Autodesk Fusion 360 part; units mm, degrees
(part 7 of 13)
  line L5346 (136.758, -112.613) -> (136.728, -112.622)
  line L5347 (137.072, -110.779) -> (137.074, -110.771)
  line L5348 (135.676, -113.181) -> (135.176, -113.181)
  line L5349 (137.072, -111.929) -> (137.072, -110.779)
  line L5350 (135.676, -111.686) -> (135.75, -111.686)
  line L5351 (137.084, -110.76) -> (137.092, -110.759)
  line L5352 (138.11, -110.76) -> (138.116, -110.765)
  line L5353 (135.176, -111.681) -> (135.676, -111.681)
  line L5354 (135.676, -111.681) -> (135.676, -111.686)
  line L5355 (138.02, -113.004) -> (137.897, -113.024)
  line L5356 (137.078, -110.765) -> (137.084, -110.76)
  line L5357 (138.12, -110.771) -> (138.122, -110.779)
  line L5358 (137.46, -110.76) -> (137.466, -110.765)
  line L5359 (137.393, -111.982) -> (137.392, -111.988)
  line L5360 (137.36, -112.041) -> (136.817, -112.585)
  line L5361 (137.392, -111.988) -> (137.375, -112.014)
  line L5362 (135.738, -113.177) -> (135.676, -113.176)
  line L5363 (136.156, -112.041) -> (136.176, -112.181)
  line L5364 (137.099, -111.949) -> (137.092, -111.949)
  line L5365 (135.996, -113.066) -> (135.875, -113.14)
  line L5366 (137.092, -110.759) -> (137.452, -110.759)
  line L5367 (135.886, -111.727) -> (136.005, -111.804)
  line L5368 (135.176, -113.181) -> (135.176, -111.681)
  line L5369 (137.472, -110.779) -> (137.472, -111.929)
  line L5370 (136.176, -112.693) -> (136.153, -112.833)
  line L5371 (136.091, -112.961) -> (135.996, -113.066)
  line L5372 (137.452, -110.759) -> (137.46, -110.76)
  line L5373 (138.116, -110.765) -> (138.12, -110.771)
  line L5374 (136.793, -112.603) -> (136.788, -112.606)
  line L5375 (135.875, -113.14) -> (135.738, -113.177)
  line L5376 (136.005, -111.804) -> (136.098, -111.912)
  line L5377 (137.074, -111.936) -> (137.072, -111.929)
  line L5378 (137.092, -111.949) -> (137.084, -111.947)
  line L5379 (137.078, -111.943) -> (137.074, -111.936)
  line L5380 (136.153, -112.833) -> (136.091, -112.961)
  line L5381 (136.176, -112.181) -> (136.176, -112.372)
  line L5382 (136.176, -112.372) -> (136.676, -112.372)
  line L5383 (141.061, -112.902) -> (140.561, -112.902)
  line L5384 (138.116, -111.943) -> (138.11, -111.947)
  line L5385 (137.773, -112.243) -> (137.797, -112.239)
  line L5386 (138.22, -112.859) -> (138.132, -112.947)
  line L5387 (138.22, -112.388) -> (138.277, -112.5)
  line L5388 (138.122, -110.779) -> (138.122, -111.929)
  line L5389 (141.061, -112.897) -> (141.061, -112.902)
  line L5390 (137.742, -111.949) -> (137.734, -111.947)
  line L5391 (141.061, -111.407) -> (141.141, -111.408)
  line L5392 (137.722, -110.779) -> (137.724, -110.771)
  line L5393 (138.77, -110.771) -> (138.772, -110.779)
  line L5394 (137.516, -112.747) -> (137.497, -112.624)
  line L5395 (137.724, -111.936) -> (137.722, -111.929)
  line L5396 (138.132, -112.947) -> (138.02, -113.004)
  line L5397 (137.661, -112.3) -> (137.773, -112.243)
  line L5398 (137.728, -111.943) -> (137.724, -111.936)
  line L5399 (138.12, -111.936) -> (138.116, -111.943)
  line L5400 (138.122, -111.929) -> (138.12, -111.936)
  line L5401 (137.573, -112.859) -> (137.516, -112.747)
  line L5402 (137.897, -113.024) -> (137.773, -113.004)
  line L5403 (138.297, -112.624) -> (138.277, -112.747)
  line L5404 (138.102, -111.949) -> (138.047, -111.949)
  line L5405 (138.277, -112.747) -> (138.22, -112.859)
  line L5406 (138.132, -112.3) -> (138.22, -112.388)
  line L5407 (138.047, -111.949) -> (138.047, -112.257)
  line L5408 (137.516, -112.5) -> (137.573, -112.388)
  line L5409 (137.573, -112.388) -> (137.661, -112.3)
  line L5410 (138.277, -112.5) -> (138.297, -112.624)
  line L5411 (141.276, -111.45) -> (141.394, -111.529)
  line L5412 (138.11, -111.947) -> (138.102, -111.949)
  line L5413 (137.773, -113.004) -> (137.661, -112.947)
  line L5414 (137.722, -111.929) -> (137.722, -110.779)
  line L5415 (137.661, -112.947) -> (137.573, -112.859)
  line L5416 (141.561, -111.902) -> (141.561, -112.402)
  line L5417 (137.734, -111.947) -> (137.728, -111.943)
  line L5418 (141.141, -111.408) -> (141.276, -111.45)
  line L5419 (137.797, -112.239) -> (137.797, -111.949)
  line L5420 (137.497, -112.624) -> (137.516, -112.5)
  line L5421 (141.061, -111.402) -> (141.061, -111.407)
  line L5422 (138.766, -110.765) -> (138.77, -110.771)
  line L5423 (138.047, -112.257) -> (138.132, -112.3)
  line L5424 (137.797, -111.949) -> (137.742, -111.949)
  line L5425 (141.265, -112.858) -> (141.129, -112.897)
  line L5426 (138.392, -111.949) -> (138.384, -111.947)
  line L5427 (137.728, -110.765) -> (137.734, -110.76)
  line L5428 (139.061, -112.414) -> (139.055, -112.413)
  line L5429 (138.772, -111.798) -> (139.142, -112.168)
  line L5430 (139.029, -112.397) -> (139.002, -112.382)
  line L5431 (141.486, -111.637) -> (141.543, -111.767)
  line L5432 (141.561, -112.408) -> (141.539, -112.548)
  line L5433 (141.56, -111.902) -> (141.561, -111.902)
  line L5434 (139.34, -112.671) -> (139.281, -112.542)
  line L5435 (139.347, -111.622) -> (139.442, -111.517)
  line L5436 (138.102, -110.759) -> (138.11, -110.76)
  line L5437 (141.56, -112.402) -> (141.561, -112.408)
  line L5438 (141.543, -111.767) -> (141.56, -111.902)
  line L5439 (139.551, -112.855) -> (139.433, -112.778)
  line L5440 (141.129, -112.897) -> (141.061, -112.897)
  line L5441 (138.76, -110.76) -> (138.766, -110.765)
  line L5442 (137.742, -110.759) -> (138.102, -110.759)
  line L5443 (141.385, -112.782) -> (141.265, -112.858)
  line L5444 (138.772, -110.779) -> (138.772, -111.798)
  line L5445 (139.055, -112.413) -> (139.029, -112.397)
  line L5446 (139.699, -111.405) -> (139.761, -111.407)
  line L5447 (140.561, -111.402) -> (141.061, -111.402)
  line L5448 (138.569, -111.949) -> (138.392, -111.949)
  line L5449 (139.068, -112.415) -> (139.064, -112.416)
  line L5450 (139.261, -112.168) -> (139.261, -111.902)
  line L5451 (140.261, -111.402) -> (140.261, -112.902)
  line L5452 (139.563, -111.443) -> (139.699, -111.405)
  line L5453 (141.394, -111.529) -> (141.486, -111.637)
  line L5454 (141.479, -112.676) -> (141.385, -112.782)
  line L5455 (137.734, -110.76) -> (137.742, -110.759)
  line L5456 (141.561, -112.402) -> (141.56, -112.402)
  line L5457 (141.539, -112.548) -> (141.479, -112.676)
  line L5458 (139.281, -112.542) -> (139.264, -112.418)
  line L5459 (139.002, -112.382) -> (138.569, -111.949)
  line L5460 (139.761, -112.902) -> (139.761, -112.897)
  line L5461 (139.09, -112.418) -> (139.068, -112.415)
  line L5462 (140.261, -112.902) -> (139.761, -112.902)
  line L5463 (138.384, -111.947) -> (138.378, -111.943)
  line L5464 (139.442, -111.517) -> (139.563, -111.443)
  line L5465 (140.561, -112.902) -> (140.561, -111.402)
  line L5466 (137.724, -110.771) -> (137.728, -110.765)
  line L5467 (139.064, -112.416) -> (139.061, -112.414)
  line L5468 (117.057, -112.867) -> (116.933, -112.886)
  line L5469 (139.761, -111.407) -> (139.761, -111.402)
  line L5470 (139.761, -112.897) -> (139.687, -112.896)
  line L5471 (117.237, -110.754) -> (117.242, -110.761)
  line L5472 (117.257, -112.722) -> (117.168, -112.81)
  line L5473 (139.261, -111.902) -> (139.261, -111.889)
  line L5474 (139.433, -112.778) -> (139.34, -112.671)
  line L5475 (117.237, -111.932) -> (117.231, -111.937)
  line L5476 (138.374, -111.936) -> (138.372, -111.929)
  line L5477 (138.378, -110.765) -> (138.384, -110.76)
  line L5478 (138.752, -110.759) -> (138.76, -110.76)
  line L5479 (139.687, -112.896) -> (139.551, -112.855)
  line L5480 (139.142, -112.168) -> (139.261, -112.168)
  line L5481 (117.314, -112.363) -> (117.333, -112.486)
  line L5482 (138.372, -111.929) -> (138.372, -110.779)
  line L5483 (139.285, -111.75) -> (139.347, -111.622)
  line L5484 (139.261, -111.889) -> (139.285, -111.75)
  line L5485 (116.698, -112.81) -> (116.61, -112.722)
  line L5486 (116.61, -112.722) -> (116.553, -112.61)
  line L5487 (117.242, -110.761) -> (117.243, -110.768)
  line L5488 (117.243, -111.918) -> (117.242, -111.926)
  line L5489 (138.374, -110.771) -> (138.378, -110.765)
  line L5490 (117.257, -112.251) -> (117.314, -112.363)
  line L5491 (117.223, -111.938) -> (117.168, -111.938)
  line L5492 (116.81, -112.867) -> (116.698, -112.81)
  line L5493 (117.231, -111.937) -> (117.223, -111.938)
  line L5494 (117.168, -111.938) -> (117.168, -112.163)
  line L5495 (117.168, -112.81) -> (117.057, -112.867)
  line L5496 (139.264, -112.418) -> (139.09, -112.418)
  line L5497 (138.384, -110.76) -> (138.392, -110.759)
  line L5498 (138.378, -111.943) -> (138.374, -111.936)
  line L5499 (138.392, -110.759) -> (138.752, -110.759)
  line L5500 (117.168, -112.163) -> (117.168, -112.163)
  line L5501 (117.243, -110.768) -> (117.243, -111.918)
  line L5502 (117.333, -112.486) -> (117.314, -112.61)
  line L5503 (139.761, -111.402) -> (140.261, -111.402)
  line L5504 (117.314, -112.61) -> (117.257, -112.722)
  line L5505 (117.168, -112.163) -> (117.257, -112.251)
  line L5506 (138.372, -110.779) -> (138.374, -110.771)
  line L5507 (117.242, -111.926) -> (117.237, -111.932)
  line L5508 (116.553, -112.61) -> (116.533, -112.486)
  line L5509 (116.933, -112.886) -> (116.81, -112.867)
  line L5510 (117.231, -110.75) -> (117.237, -110.754)
  line L5511 (137.406, -96.1939) -> (137.421, -96.2704)
  line L5512 (137.362, -96.9618) -> (137.297, -97.0052)
  line L5513 (116.856, -110.75) -> (116.863, -110.748)
  line L5514 (116.918, -112.089) -> (116.918, -111.938)
  line L5515 (136.636, -96.1939) -> (136.679, -96.129)
  line L5516 (116.553, -112.363) -> (116.61, -112.251)
  line L5517 (137.221, -96.0704) -> (137.297, -96.0856)
  line L5518 (116.856, -111.937) -> (116.849, -111.932)
  line L5519 (136.569, -97.9424) -> (136.55, -98.066)
  line L5520 (136.493, -97.7073) -> (136.55, -97.8188)
  line L5521 (135.609, -96.129) -> (135.652, -96.1939)
  line L5522 (136.679, -96.129) -> (136.744, -96.0856)
  line L5523 (137.421, -96.8204) -> (137.406, -96.8969)
  line L5524 (116.863, -110.748) -> (117.223, -110.748)
  line L5525 (116.698, -112.163) -> (116.81, -112.106)
  line L5526 (116.845, -111.926) -> (116.843, -111.918)
  line L5527 (137.297, -96.0856) -> (137.362, -96.129)
  line L5528 (135.667, -96.2704) -> (135.667, -96.7686)
  line L5529 (135.544, -96.0856) -> (135.609, -96.129)
  line L5530 (136.144, -97.2454) -> (136.621, -96.7686)
  line L5531 (116.845, -110.761) -> (116.849, -110.754)
  line L5532 (116.843, -110.768) -> (116.845, -110.761)
  line L5533 (116.849, -110.754) -> (116.856, -110.75)
  line L5534 (116.849, -111.932) -> (116.845, -111.926)
  line L5535 (116.843, -111.918) -> (116.843, -110.768)
  line L5536 (117.223, -110.748) -> (117.231, -110.75)
  line L5537 (135.667, -96.7686) -> (136.144, -97.2454)
  line L5538 (136.744, -96.0856) -> (136.821, -96.0704)
  line L5539 (136.821, -96.0704) -> (137.221, -96.0704)
  line L5540 (136.55, -97.8188) -> (136.569, -97.9424)
  line L5541 (136.621, -96.2704) -> (136.636, -96.1939)
  line L5542 (116.918, -111.938) -> (116.863, -111.938)
  line L5543 (116.533, -112.486) -> (116.553, -112.363)
  line L5544 (136.046, -98.3228) -> (135.993, -98.2958)
  line L5545 (116.61, -112.251) -> (116.698, -112.163)
  line L5546 (136.169, -98.3424) -> (136.046, -98.3228)
  line L5547 (135.993, -98.2958) -> (134.581, -99.7072)
  line L5548 (136.74, -97.0026) -> (136.294, -97.4486)
  line L5549 (136.405, -97.6188) -> (136.493, -97.7073)
  line L5550 (116.81, -112.106) -> (116.918, -112.089)
  line L5551 (136.621, -96.7686) -> (136.621, -96.2704)
  line L5552 (116.863, -111.938) -> (116.856, -111.937)
  line L5553 (135.652, -96.1939) -> (135.667, -96.2704)
  line L5554 (137.421, -96.2704) -> (137.421, -96.8204)
  line L5555 (127.249, -111.914) -> (127.248, -111.916)
  line L5556 (134.558, -99.7248) -> (134.553, -99.7287)
  line L5557 (130.089, -99.7387) -> (130.063, -99.722)
  line L5558 (130.063, -99.722) -> (130.052, -99.7158)
  line L5559 (127.252, -111.887) -> (127.249, -111.909)
  line L5560 (126.666, -112.852) -> (126.543, -112.871)
  line L5561 (134.493, -99.7438) -> (130.124, -99.7438)
  line L5562 (130.124, -99.7438) -> (130.102, -99.7406)
  line L5563 (126.778, -112.795) -> (126.666, -112.852)
  line L5564 (136.294, -97.4486) -> (136.294, -97.5627)
  line L5565 (136.821, -97.0204) -> (136.744, -97.0052)
  line L5566 (136.405, -98.266) -> (136.293, -98.3228)
  line L5567 (134.564, -99.7205) -> (134.561, -99.724)
  line L5568 (134.553, -99.7287) -> (134.523, -99.7351)
  line L5569 (137.297, -97.0052) -> (137.221, -97.0204)
  line L5570 (137.362, -96.129) -> (137.406, -96.1939)
  line L5571 (136.294, -97.5627) -> (136.405, -97.6188)
  line L5572 (130.098, -99.7409) -> (130.095, -99.7396)
  line L5573 (134.581, -99.7072) -> (134.564, -99.7205)
  line L5574 (127.243, -107.93) -> (127.252, -107.959)
  line L5575 (127.233, -107.894) -> (127.237, -107.9)
  line L5576 (126.896, -112.295) -> (126.923, -112.348)
  line L5577 (126.923, -112.348) -> (126.943, -112.471)
  line L5578 (127.23, -111.948) -> (127.215, -111.975)
  line L5579 (126.943, -112.471) -> (126.923, -112.595)
  line L5580 (127.215, -111.975) -> (126.896, -112.295)
  line L5581 (127.229, -107.889) -> (127.232, -107.892)
  line L5582 (127.247, -111.923) -> (127.23, -111.948)
  line L5583 (136.293, -98.3228) -> (136.169, -98.3424)
  line L5584 (130.102, -99.7406) -> (130.098, -99.7409)
  line L5585 (137.221, -97.0204) -> (136.821, -97.0204)
  line L5586 (136.744, -97.0052) -> (136.74, -97.0026)
  line L5587 (134.561, -99.724) -> (134.558, -99.7248)
  line L5588 (134.523, -99.7351) -> (134.493, -99.7438)
  line L5589 (126.923, -112.595) -> (126.866, -112.706)
  line L5590 (136.55, -98.066) -> (136.493, -98.1775)
  line L5591 (137.406, -96.8969) -> (137.362, -96.9618)
  line L5592 (126.654, -103.113) -> (126.654, -107.31)
  line L5593 (127.248, -111.916) -> (127.247, -111.923)
  line L5594 (130.052, -99.7158) -> (126.654, -103.113)
  line L5595 (130.095, -99.7396) -> (130.089, -99.7387)
  line L5596 (136.493, -98.1775) -> (136.405, -98.266)
  line L5597 (127.237, -107.9) -> (127.243, -107.93)
  line L5598 (126.654, -107.31) -> (127.215, -107.871)
  line L5599 (130.031, -99.4236) -> (130.057, -99.4179)
  line L5600 (135.067, -96.0704) -> (135.467, -96.0704)
  line L5601 (135.467, -96.0704) -> (135.544, -96.0856)
  line L5602 (126.866, -112.706) -> (126.778, -112.795)
  line L5603 (129.997, -99.4308) -> (130.004, -99.4254)
  line L5604 (127.215, -107.871) -> (127.229, -107.889)
  line L5605 (126.219, -112.236) -> (126.308, -112.148)
  line L5606 (129.96, -99.4542) -> (129.988, -99.4327)
  line L5607 (126.543, -112.871) -> (126.419, -112.852)
  line L5608 (126.162, -112.595) -> (126.143, -112.471)
  line L5609 (126.308, -112.148) -> (126.419, -112.091)
  line L5610 (126.427, -107.432) -> (126.424, -107.429)
  line L5611 (126.423, -107.426) -> (126.419, -107.421)
  line L5612 (126.441, -107.45) -> (126.427, -107.432)
  line L5613 (126.407, -103.035) -> (126.408, -103.032)
  line L5614 (126.424, -107.429) -> (126.423, -107.426)
  line L5615 (126.162, -112.348) -> (126.219, -112.236)
  line L5616 (126.404, -107.361) -> (126.404, -103.062)
  line L5617 (126.308, -112.795) -> (126.219, -112.706)
  line L5618 (126.419, -112.852) -> (126.308, -112.795)
  line L5619 (126.407, -103.04) -> (126.407, -103.035)
  line L5620 (126.408, -103.032) -> (126.409, -103.026)
  line L5621 (126.666, -112.091) -> (126.719, -112.118)
  line L5622 (126.413, -107.391) -> (126.404, -107.361)
  line L5623 (126.426, -103) -> (126.441, -102.973)
  line L5624 (126.419, -107.421) -> (126.413, -107.391)
  line L5625 (130.004, -99.4254) -> (130.031, -99.4236)
  line L5626 (127.002, -108.011) -> (126.441, -107.45)
  line L5627 (127.232, -107.892) -> (127.233, -107.894)
  line L5628 (126.143, -112.471) -> (126.162, -112.348)
  line L5629 (126.404, -103.062) -> (126.407, -103.04)
  line L5630 (126.441, -102.973) -> (129.96, -99.4542)
  line L5631 (127.002, -111.835) -> (127.002, -108.011)
  line L5632 (126.719, -112.118) -> (127.002, -111.835)
  line L5633 (127.249, -111.909) -> (127.249, -111.914)
  line L5634 (126.409, -103.026) -> (126.426, -103)
  line L5635 (126.419, -112.091) -> (126.543, -112.071)
  line L5636 (127.252, -107.959) -> (127.252, -111.887)
  line L5637 (126.219, -112.706) -> (126.162, -112.595)
  line L5638 (126.543, -112.071) -> (126.666, -112.091)
  line L5639 (129.988, -99.4327) -> (129.997, -99.4308)
  line L5640 (129.697, -96.0196) -> (130.097, -96.0196)
  line L5641 (134.867, -96.8204) -> (134.867, -96.2704)
  line L5642 (130.066, -99.4211) -> (130.075, -99.4205)
  line L5643 (135.846, -97.7073) -> (135.934, -97.6188)
  line L5644 (130.238, -96.0782) -> (130.281, -96.1431)
  line L5645 (130.123, -99.4426) -> (130.128, -99.4499)
  line L5646 (130.238, -96.911) -> (130.173, -96.9544)
  line L5647 (135.544, -97.0052) -> (135.467, -97.0204)
  line L5648 (130.128, -99.4499) -> (130.136, -99.4542)
  line L5649 (135.816, -98.119) -> (135.789, -98.066)
  line L5650 (135.769, -97.9424) -> (135.789, -97.8188)
  line L5651 (130.097, -96.0196) -> (130.173, -96.0348)
  line L5652 (129.497, -96.2196) -> (129.512, -96.1431)
  line L5653 (130.016, -98.4595) -> (130, -98.4854)
  line L5654 (135.548, -97.0026) -> (135.544, -97.0052)
  line L5655 (135.467, -97.0204) -> (135.067, -97.0204)
  line L5656 (134.882, -96.1939) -> (134.926, -96.129)
  line L5657 (134.926, -96.9618) -> (134.882, -96.8969)
  line L5658 (130.075, -99.4205) -> (130.098, -99.4333)
  line L5659 (134.882, -96.8969) -> (134.867, -96.8204)
  line L5660 (130.176, -99.4938) -> (134.441, -99.4938)
  line L5661 (129.772, -96.9696) -> (129.697, -96.9696)
  line L5662 (134.991, -96.0856) -> (135.067, -96.0704)
  line L5663 (134.867, -96.2704) -> (134.882, -96.1939)
  line L5664 (135.067, -97.0204) -> (134.991, -97.0052)
  line L5665 (135.789, -97.8188) -> (135.846, -97.7073)
  line L5666 (134.991, -97.0052) -> (134.926, -96.9618)
  line L5667 (135.934, -97.6188) -> (136.044, -97.5627)
  line L5668 (130.098, -99.4333) -> (130.123, -99.4426)
  line L5669 (130.173, -96.9544) -> (130.097, -96.9696)
  line L5670 (135.789, -98.066) -> (135.769, -97.9424)
  line L5671 (129.697, -96.9696) -> (129.62, -96.9544)
  line L5672 (130.136, -99.4542) -> (130.176, -99.4938)
  line L5673 (136.044, -97.4994) -> (135.548, -97.0026)
  line L5674 (136.044, -97.5627) -> (136.044, -97.4994)
  line L5675 (129.497, -96.7696) -> (129.497, -96.2196)
  line L5676 (130.057, -99.4179) -> (130.066, -99.4211)
  line L5677 (134.926, -96.129) -> (134.991, -96.0856)
  line L5678 (134.441, -99.4938) -> (135.816, -98.119)
  line L5679 (129.62, -96.0348) -> (129.697, -96.0196)
  line L5680 (130.297, -96.2196) -> (130.297, -96.7696)
  line L5681 (130.281, -96.8461) -> (130.238, -96.911)
  line L5682 (130.297, -96.7696) -> (130.281, -96.8461)
  line L5683 (125.972, -108.013) -> (125.958, -107.995)
  line L5684 (130.022, -96.9696) -> (130.022, -98.424)
  line L5685 (126.318, -110.113) -> (126.422, -110.166)
  line L5686 (126.299, -107.99) -> (126.299, -107.993)
  line L5687 (125.864, -110.725) -> (125.807, -110.614)
  line L5688 (125.95, -107.984) -> (125.944, -107.954)
  line L5689 (126.568, -110.614) -> (126.511, -110.725)
  line L5690 (129.985, -98.5124) -> (126.185, -102.312)
  line L5691 (126.185, -107.873) -> (126.282, -107.969)
  line L5692 (126.422, -110.814) -> (126.311, -110.87)
  line L5693 (126.422, -110.166) -> (126.511, -110.255)
  line L5694 (129.555, -96.911) -> (129.512, -96.8461)
  line L5695 (126.295, -107.987) -> (126.299, -107.99)
  line L5696 (129.512, -96.1431) -> (129.555, -96.0782)
  line L5697 (125.954, -107.989) -> (125.95, -107.984)
  line L5698 (125.952, -110.166) -> (126.064, -110.11)
  line L5699 (130.097, -96.9696) -> (130.022, -96.9696)
  line L5700 (129.512, -96.8461) -> (129.497, -96.7696)
  line L5701 (129.62, -96.9544) -> (129.555, -96.911)
  line L5702 (129.555, -96.0782) -> (129.62, -96.0348)
  line L5703 (130, -98.4854) -> (129.985, -98.5124)
  line L5704 (130.019, -98.4506) -> (130.017, -98.4531)
  line L5705 (130.173, -96.0348) -> (130.238, -96.0782)
  line L5706 (130.281, -96.1431) -> (130.297, -96.2196)
  line L5707 (126.064, -110.87) -> (125.952, -110.814)
  line L5708 (126.068, -110.109) -> (126.068, -108.11)
  line L5709 (130.022, -98.424) -> (130.018, -98.446)
  line L5710 (130.018, -98.446) -> (130.019, -98.4506)
  line L5711 (126.185, -102.312) -> (126.185, -107.873)
  line L5712 (126.282, -107.969) -> (126.295, -107.987)
  line L5713 (130.017, -98.4531) -> (130.016, -98.4595)
  line L5714 (125.864, -110.255) -> (125.952, -110.166)
  line L5715 (125.944, -107.954) -> (125.935, -107.925)
  line L5716 (125.807, -110.614) -> (125.787, -110.49)
  line L5717 (126.511, -110.255) -> (126.568, -110.366)
  line L5718 (124.136, -94.1898) -> (124.225, -94.2783)
  line L5719 (112.559, -93.01) -> (112.464, -93.1343)
  line L5720 (113.488, -91.438) -> (112.54, -92.3858)
  line L5721 (110.74, -97.1174) -> (110.597, -97.203)
  line L5722 (123.901, -94.9134) -> (123.778, -94.8938)
  line L5723 (110.412, -95.7843) -> (110.458, -95.7898)
  line L5724 (123.521, -94.637) -> (123.501, -94.5134)
  line L5725 (124.225, -94.2783) -> (124.272, -94.3718)
  line L5726 (111.037, -96.5409) -> (111.013, -96.7065)
  line L5727 (110.954, -96.8628) -> (110.861, -97.0021)
  line L5728 (111.037, -96.52) -> (111.037, -96.5409)
  line L5729 (124.025, -94.8938) -> (123.901, -94.9134)
  line L5730 (124.337, -94.6297) -> (124.308, -94.6384)
  line L5731 (109.615, -96.1865) -> (109.706, -96.046)
  line L5732 (112.339, -93.2296) -> (112.195, -93.2896)
  line L5733 (123.666, -94.1898) -> (123.778, -94.133)
  line L5734 (124.225, -94.7485) -> (124.136, -94.837)
  line L5735 (123.521, -94.3898) -> (123.578, -94.2783)
  line L5736 (111.884, -93.2896) -> (111.739, -93.2296)
  line L5737 (111.739, -93.2296) -> (111.715, -93.211)
  line L5738 (111.018, -96.3538) -> (111.037, -96.52)
  line L5739 (112.195, -93.2896) -> (112.039, -93.31)
  line L5740 (123.501, -94.5134) -> (123.521, -94.3898)
  line L5741 (124.281, -94.6384) -> (124.225, -94.7485)
  line L5742 (112.619, -92.5547) -> (112.639, -92.71)
  line L5743 (123.778, -94.8938) -> (123.666, -94.837)
  line L5744 (124.308, -94.6384) -> (124.281, -94.6384)
  line L5745 (124.025, -94.133) -> (124.136, -94.1898)
  line L5746 (111.013, -96.7065) -> (110.954, -96.8628)
  line L5747 (123.578, -94.2783) -> (123.666, -94.1898)
  line L5748 (110.963, -96.1959) -> (111.018, -96.3538)
  line L5749 (123.901, -94.1134) -> (124.025, -94.133)
  line L5750 (112.464, -93.1343) -> (112.339, -93.2296)
  line L5751 (110.412, -94.5144) -> (110.412, -95.7843)
  line L5752 (124.272, -94.3718) -> (125.199, -93.4456)
  line L5753 (110.757, -95.9355) -> (110.875, -96.0541)
  line L5754 (110.861, -97.0021) -> (110.74, -97.1174)
  line L5755 (110.438, -97.2547) -> (110.271, -97.2698)
  line L5756 (111.715, -93.211) -> (110.412, -94.5144)
  line L5757 (110.875, -96.0541) -> (110.963, -96.1959)
  line L5758 (112.039, -93.31) -> (111.884, -93.2896)
  line L5759 (123.778, -94.133) -> (123.901, -94.1134)
  line L5760 (110.616, -95.8459) -> (110.757, -95.9355)
  line L5761 (124.136, -94.837) -> (124.025, -94.8938)
  line L5762 (123.666, -94.837) -> (123.578, -94.7485)
  line L5763 (110.458, -95.7898) -> (110.616, -95.8459)
  line L5764 (110.597, -97.203) -> (110.438, -97.2547)
  line L5765 (110.271, -97.2698) -> (110.105, -97.2477)
  line L5766 (109.949, -97.1894) -> (109.809, -97.0979)
  line L5767 (109.809, -97.0979) -> (109.693, -96.9776)
  line L5768 (109.553, -96.6759) -> (109.537, -96.5095)
  line L5769 (109.693, -96.9776) -> (109.606, -96.8346)
  line L5770 (109.537, -96.5095) -> (109.558, -96.3436)
  line L5771 (110.105, -97.2477) -> (109.949, -97.1894)
  line L5772 (109.558, -96.3436) -> (109.615, -96.1865)
  line L5773 (109.606, -96.8346) -> (109.553, -96.6759)
  line L5774 (113.348, -91.2246) -> (113.366, -91.2113)
  line L5775 (112.039, -92.11) -> (112.195, -92.1304)
  line L5776 (128.831, -106.298) -> (128.331, -106.298)
  line L5777 (121.753, -109.441) -> (121.699, -109.359)
  line L5778 (128.331, -106.298) -> (128.331, -106.293)
  line L5779 (123.225, -107.8) -> (123.228, -107.801)
  line L5780 (123.194, -107.807) -> (123.225, -107.8)
  line L5781 (128.306, -106.292) -> (127.638, -106.96)
  line L5782 (123.127, -107.836) -> (123.156, -107.815)
  line L5783 (128.331, -106.293) -> (128.306, -106.292)
  line L5784 (127.853, -105.151) -> (127.913, -105.023)
  line L5785 (123.16, -107.814) -> (123.162, -107.811)
  line L5786 (128.263, -104.802) -> (128.331, -104.803)
  line L5787 (126.874, -107.185) -> (126.854, -107.061)
  line L5788 (127.378, -107.441) -> (127.254, -107.461)
  line L5789 (126.854, -107.061) -> (126.874, -106.937)
  line L5790 (127.019, -106.737) -> (127.13, -106.681)
  line L5791 (128.007, -104.917) -> (128.127, -104.841)
  line L5792 (127.85, -105.932) -> (127.832, -105.798)
  line L5793 (127.13, -107.441) -> (127.019, -107.385)
  line L5794 (127.831, -105.291) -> (127.853, -105.151)
  line L5795 (139.012, -96.129) -> (139.056, -96.1939)
  line L5796 (127.831, -105.798) -> (127.831, -105.298)
  line L5797 (138.947, -96.0856) -> (139.012, -96.129)
  line L5798 (127.13, -106.681) -> (127.254, -106.661)
  line L5799 (127.254, -106.661) -> (127.355, -106.677)
  line L5800 (128.127, -104.841) -> (128.263, -104.802)
  line L5801 (126.874, -106.937) -> (126.93, -106.826)
  line L5802 (126.93, -106.826) -> (127.019, -106.737)
  line L5803 (126.93, -107.296) -> (126.874, -107.185)
  line L5804 (127.254, -107.461) -> (127.13, -107.441)
  line L5805 (127.355, -106.677) -> (127.936, -106.096)
  line L5806 (127.907, -106.062) -> (127.85, -105.932)
  line L5807 (128.331, -104.803) -> (128.331, -104.798)
  line L5808 (127.936, -106.096) -> (127.907, -106.062)
  line L5809 (127.832, -105.298) -> (127.831, -105.291)
  line L5810 (128.331, -104.798) -> (128.831, -104.798)
  line L5811 (127.913, -105.023) -> (128.007, -104.917)
  line L5812 (127.489, -107.385) -> (127.378, -107.441)
  line L5813 (127.831, -105.298) -> (127.832, -105.298)
  line L5814 (127.832, -105.798) -> (127.831, -105.798)
  line L5815 (127.019, -107.385) -> (126.93, -107.296)
  line L5816 (128.831, -104.798) -> (128.831, -106.298)
  line L5817 (140.174, -99.6955) -> (140.112, -99.7023)
  line L5818 (139.157, -97.4727) -> (139.171, -97.4665)
  line L5819 (141.184, -98.7889) -> (141.184, -99.5695)
  line L5820 (141.164, -99.6376) -> (141.11, -99.6841)
  line L5821 (136.56, -106.503) -> (136.54, -106.483)
  line L5822 (138.931, -97.5267) -> (138.935, -97.5277)
  line L5823 (139.505, -97.1785) -> (139.575, -97.1665)
  line L5824 (138.925, -97.5103) -> (138.929, -97.5255)
  line L5825 (139.427, -97.2658) -> (139.436, -97.254)
  line L5826 (139.071, -96.8204) -> (139.056, -96.8969)
  line L5827 (136.612, -106.552) -> (136.562, -106.506)
  line L5828 (138.763, -106.953) -> (137.037, -106.93)
  line L5829 (139.714, -100.156) -> (139.714, -106.092)
  line L5830 (141.11, -99.6841) -> (141.058, -99.6955)
  line L5831 (138.935, -97.5277) -> (138.994, -97.5223)
  line L5832 (136.528, -106.473) -> (136.501, -106.448)
  line L5833 (139.72, -106.154) -> (139.772, -106.291)
  line L5834 (139.866, -106.413) -> (139.872, -106.419)
  line L5835 (139.453, -97.2264) -> (139.505, -97.1785)
  line L5836 (139.859, -106.407) -> (139.866, -106.413)
  line L5837 (136.501, -106.448) -> (136.495, -106.443)
  line L5838 (139.904, -106.466) -> (139.909, -106.537)
  line L5839 (139.056, -96.8969) -> (139.012, -96.9618)
  line L5840 (137.037, -106.93) -> (136.97, -106.91)
  line L5841 (139.487, -106.959) -> (139.459, -106.962)
  line L5842 (139.64, -97.1943) -> (139.65, -97.2026)
  line L5843 (138.925, -97.0097) -> (138.925, -97.5103)
  line L5844 (141.058, -99.6955) -> (140.174, -99.6955)
  line L5845 (139.459, -106.962) -> (138.763, -106.953)
  line L5846 (139.056, -96.1939) -> (139.071, -96.2704)
  line L5847 (138.994, -97.5223) -> (139.007, -97.5197)
  line L5848 (141.184, -99.5695) -> (141.164, -99.6376)
  line L5849 (139.65, -97.2026) -> (141.147, -98.6998)
  line L5850 (139.171, -97.4665) -> (139.304, -97.3856)
  line L5851 (141.181, -98.7621) -> (141.184, -98.7889)
  line L5852 (139.316, -97.3763) -> (139.427, -97.2658)
  line L5853 (139.975, -99.7534) -> (139.859, -99.8407)
  line L5854 (139.87, -106.421) -> (139.904, -106.466)
  line L5855 (139.007, -97.5197) -> (139.157, -97.4727)
  line L5856 (138.947, -97.0052) -> (138.925, -97.0097)
  line L5857 (139.909, -106.537) -> (139.875, -106.599)
  line L5858 (139.875, -106.599) -> (139.55, -106.925)
  line L5859 (139.012, -96.9618) -> (138.947, -97.0052)
  line L5860 (139.575, -97.1665) -> (139.64, -97.1943)
  line L5861 (139.304, -97.3856) -> (139.316, -97.3763)
  line L5862 (139.859, -99.8407) -> (139.772, -99.9573)
  line L5863 (139.436, -97.254) -> (139.453, -97.2264)
  line L5864 (136.95, -106.894) -> (136.624, -106.567)
  line L5865 (139.872, -106.419) -> (139.87, -106.421)
  line L5866 (136.616, -106.559) -> (136.612, -106.552)
  line L5867 (136.624, -106.567) -> (136.616, -106.559)
  line L5868 (139.72, -100.094) -> (139.714, -100.156)
  line L5869 (136.54, -106.483) -> (136.537, -106.481)
  line L5870 (139.714, -106.092) -> (139.72, -106.154)
  line L5871 (139.772, -106.291) -> (139.859, -106.407)
  line L5872 (136.562, -106.506) -> (136.56, -106.503)
  line L5873 (139.55, -106.925) -> (139.487, -106.959)
  line L5874 (138.929, -97.5255) -> (138.931, -97.5267)
  line L5875 (136.97, -106.91) -> (136.95, -106.894)
  line L5876 (139.772, -99.9573) -> (139.72, -100.094)
  line L5877 (136.537, -106.481) -> (136.528, -106.473)
  line L5878 (139.071, -96.2704) -> (139.071, -96.8204)
  line L5879 (141.147, -98.6998) -> (141.181, -98.7621)
  line L5880 (140.112, -99.7023) -> (139.975, -99.7534)
  line L5881 (136.62, -98.7362) -> (136.626, -98.7335)
  line L5882 (136.626, -98.7335) -> (136.781, -98.6213)
  line L5883 (135.375, -99.8407) -> (135.372, -99.8383)
  line L5884 (136.404, -106.392) -> (136.394, -106.387)
  line L5885 (135.339, -99.7782) -> (135.336, -99.7517)
  line L5886 (136.495, -106.443) -> (136.488, -106.439)
  line L5887 (136.084, -106.326) -> (135.631, -106.326)
  line L5888 (136.298, -106.346) -> (136.29, -106.345)
  line L5889 (136.438, -106.407) -> (136.404, -106.392)
  line L5890 (136.62, -98.7362) -> (136.62, -98.7362)
  line L5891 (136.781, -98.6213) -> (136.796, -98.604)
  line L5892 (136.796, -98.604) -> (136.904, -98.4843)
  line L5893 (136.132, -106.322) -> (136.096, -106.325)
  line L5894 (136.317, -106.354) -> (136.305, -106.349)
  line L5895 (136.254, -106.339) -> (136.243, -106.337)
  line L5896 (135.336, -99.7517) -> (135.336, -99.7238)
  line L5897 (136.16, -106.324) -> (136.148, -106.322)
  line L5898 (135.521, -100.156) -> (135.514, -100.094)
  line L5899 (136.335, -106.361) -> (136.317, -106.354)
  line L5900 (136.18, -106.326) -> (136.16, -106.324)
  line L5901 (136.394, -106.387) -> (136.355, -106.366)
  line L5902 (136.148, -106.322) -> (136.14, -106.321)
  line L5903 (135.336, -99.7238) -> (135.356, -99.6557)
  line L5904 (136.182, -98.8538) -> (136.209, -98.8509)
  line L5905 (136.461, -106.422) -> (136.457, -106.419)
  line L5906 (136.438, -106.407) -> (136.438, -106.407)
  line L5907 (136.096, -106.325) -> (136.084, -106.326)
  line L5908 (136.305, -106.349) -> (136.305, -106.349)
  line L5909 (135.514, -100.094) -> (135.463, -99.9573)
  line L5910 (135.463, -99.9573) -> (135.375, -99.8407)
  line L5911 (136.488, -106.439) -> (136.478, -106.433)
  line L5912 (136.457, -106.419) -> (136.445, -106.41)
  line L5913 (136.488, -106.439) -> (136.488, -106.439)
  line L5914 (136.29, -106.345) -> (136.29, -106.345)
  line L5915 (136.305, -106.349) -> (136.298, -106.346)
  line L5916 (136.355, -106.366) -> (136.335, -106.361)
  line L5917 (135.356, -99.6557) -> (135.373, -99.6344)
  line L5918 (135.373, -99.6344) -> (136.12, -98.8878)
  line L5919 (135.51, -106.17) -> (135.509, -106.169)
  line L5920 (135.507, -106.182) -> (135.51, -106.17)
  line L5921 (136.265, -98.8509) -> (136.271, -98.8495)
  line L5922 (136.12, -98.8878) -> (136.182, -98.8538)
  line L5923 (136.271, -98.8495) -> (136.271, -98.8495)
  line L5924 (136.14, -106.321) -> (136.132, -106.322)
  line L5925 (135.631, -106.326) -> (135.563, -106.306)
  line L5926 (136.29, -106.345) -> (136.254, -106.339)
  line L5927 (135.517, -106.252) -> (135.507, -106.182)
  line L5928 (136.243, -106.337) -> (136.208, -106.328)
  line L5929 (136.209, -98.8509) -> (136.265, -98.8509)
  line L5930 (135.514, -106.154) -> (135.521, -106.092)
  line L5931 (135.372, -99.8383) -> (135.339, -99.7782)
  line L5932 (136.271, -98.8495) -> (136.358, -98.831)
  line L5933 (135.509, -106.169) -> (135.511, -106.162)
  line L5934 (135.521, -106.092) -> (135.521, -100.156)
  line L5935 (136.358, -98.831) -> (136.452, -98.8112)
  line L5936 (136.445, -106.41) -> (136.438, -106.407)
  line L5937 (136.452, -98.8112) -> (136.469, -98.8035)
  line L5938 (136.208, -106.328) -> (136.2, -106.326)
  line L5939 (136.478, -106.433) -> (136.461, -106.422)
  line L5940 (135.563, -106.306) -> (135.517, -106.252)
  line L5941 (136.469, -98.8035) -> (136.62, -98.7362)
  line L5942 (136.2, -106.326) -> (136.18, -106.326)
  line L5943 (136.208, -106.328) -> (136.208, -106.328)
  line L5944 (135.511, -106.162) -> (135.514, -106.154)
  line L5945 (137.89, -97.2572) -> (137.935, -97.2862)
  line L5946 (138.286, -96.1939) -> (138.329, -96.129)
  line L5947 (137.083, -97.9424) -> (137.073, -97.8497)
  line L5948 (138.329, -96.129) -> (138.394, -96.0856)
  line L5949 (138.471, -96.0704) -> (138.871, -96.0704)
  line L5950 (137.757, -97.2862) -> (137.819, -97.2521)
  line L5951 (137.819, -97.2521) -> (137.89, -97.2572)
  line L5952 (137.164, -97.5289) -> (137.277, -97.5289)
  line L5953 (137.661, -97.382) -> (137.757, -97.2862)
  line L5954 (137.063, -97.7525) -> (137.044, -97.6938)
  line L5955 (137.044, -97.6938) -> (137.042, -97.6229)
  line L5956 (138.171, -97.4665) -> (138.185, -97.4727)
  line L5957 (108.4, -104.881) -> (108.481, -104.935)
  line L5958 (108.535, -105.017) -> (108.554, -105.112)
  line L5959 (137.064, -98.1181) -> (137.082, -97.949)
  line L5960 (137.001, -98.3197) -> (137.001, -98.3197)
  line L5961 (137.351, -97.5222) -> (137.359, -97.5197)
  line L5962 (136.904, -98.4843) -> (136.908, -98.4793)
  line L5963 (137.28, -97.5286) -> (137.28, -97.5286)
  line L5964 (137.063, -98.1323) -> (137.064, -98.1181)
  line L5965 (137.082, -97.949) -> (137.083, -97.9424)
  line L5966 (137.277, -97.5289) -> (137.28, -97.5286)
  line L5967 (137.514, -97.4709) -> (137.661, -97.382)
  line L5968 (137.142, -97.5307) -> (137.164, -97.5289)
  line L5969 (138.394, -97.0052) -> (138.329, -96.9618)
  line L5970 (138.271, -96.2704) -> (138.286, -96.1939)
  line L5971 (138.334, -97.5197) -> (138.347, -97.5223)
  line L5972 (137.316, -97.5254) -> (137.351, -97.5222)
  line L5973 (137.004, -98.314) -> (137.063, -98.1323)
  line L5974 (137.359, -97.5197) -> (137.507, -97.4731)
  line L5975 (137.001, -98.3197) -> (137.004, -98.314)
  line L5976 (137.935, -97.2862) -> (138.025, -97.3763)
  line L5977 (138.415, -97.5225) -> (138.417, -97.5149)
  line L5978 (138.271, -96.8204) -> (138.271, -96.2704)
  line L5979 (136.968, -98.3764) -> (137.001, -98.3197)
  line L5980 (137.079, -97.5621) -> (137.142, -97.5307)
  line L5981 (138.414, -97.5239) -> (138.415, -97.5225)
  line L5982 (138.037, -97.3856) -> (138.171, -97.4665)
  line L5983 (137.064, -97.759) -> (137.064, -97.759)
  line L5984 (138.417, -97.0097) -> (138.394, -97.0052)
  line L5985 (137.073, -97.8497) -> (137.064, -97.759)
  line L5986 (138.871, -96.0704) -> (138.947, -96.0856)
  line L5987 (138.394, -96.0856) -> (138.471, -96.0704)
  line L5988 (136.904, -98.4843) -> (136.904, -98.4843)
  line L5989 (138.402, -97.5273) -> (138.414, -97.5239)
  line L5990 (137.507, -97.4731) -> (137.507, -97.4731)
  line L5991 (137.28, -97.5286) -> (137.316, -97.5254)
  line L5992 (138.329, -96.9618) -> (138.286, -96.8969)
  line L5993 (105.98, -103.752) -> (106.094, -103.837)
  line L5994 (106.094, -103.837) -> (107.119, -104.862)
  line L5995 (137.042, -97.6229) -> (137.079, -97.5621)
  line L5996 (138.025, -97.3763) -> (138.037, -97.3856)
  line L5997 (107.119, -104.862) -> (108.304, -104.862)
  line L5998 (137.507, -97.4731) -> (137.514, -97.4709)
  line L5999 (136.908, -98.4793) -> (136.968, -98.3764)
  line L6000 (138.417, -97.5149) -> (138.417, -97.0097)
  line L6001 (108.481, -104.935) -> (108.535, -105.017)
  line L6002 (138.286, -96.8969) -> (138.271, -96.8204)
  line L6003 (138.347, -97.5223) -> (138.402, -97.5273)
  line L6004 (108.304, -104.862) -> (108.4, -104.881)
  line L6005 (105.848, -103.702) -> (105.98, -103.752)
  line L6006 (108.554, -105.112) -> (108.554, -105.762)
  line L6007 (137.064, -97.759) -> (137.063, -97.7525)
  line L6008 (138.185, -97.4727) -> (138.334, -97.5197)
  line L6009 (108.304, -106.012) -> (107.774, -106.012)
  line L6010 (108.481, -105.939) -> (108.4, -105.993)
  line L6011 (103.168, -106.852) -> (101.073, -106.852)
  line L6012 (103.457, -106.951) -> (103.406, -106.944)
  line L6013 (103.638, -105.934) -> (103.658, -105.951)
  line L6014 (103.223, -106.89) -> (103.207, -106.878)
  line L6015 (106.897, -106.873) -> (106.878, -106.881)
  line L6016 (106.729, -106.941) -> (106.678, -106.944)
  line L6017 (103.317, -106.93) -> (103.271, -106.908)
  line L6018 (103.489, -105.87) -> (103.509, -105.873)
  line L6019 (103.854, -103.011) -> (103.897, -103.076)
  line L6020 (103.913, -103.553) -> (103.897, -103.629)
  line L6021 (105.342, -103.889) -> (105.443, -103.789)
  line L6022 (106.814, -106.91) -> (106.768, -106.931)
  line L6023 (106.981, -106.805) -> (106.977, -106.809)
  line L6024 (103.897, -103.629) -> (103.854, -103.694)
  line L6025 (103.509, -105.873) -> (103.556, -105.895)
  line L6026 (103.603, -105.913) -> (103.619, -105.925)
  line L6027 (103.271, -106.908) -> (103.223, -106.89)
  line L6028 (106.607, -105.765) -> (105.387, -104.544)
  line L6029 (105.443, -103.789) -> (105.568, -103.722)
  line L6030 (105.242, -104.151) -> (105.273, -104.012)
  line L6031 (96.4732, -106.902) -> (96.4732, -105.802)
  line L6032 (105.706, -103.692) -> (105.848, -103.702)
  line L6033 (106.42, -105.951) -> (106.607, -105.765)
  line L6034 (106.748, -106.934) -> (106.729, -106.941)
  line L6035 (103.188, -106.869) -> (103.168, -106.852)
  line L6036 (106.678, -106.944) -> (106.627, -106.951)
  line L6037 (105.299, -104.426) -> (105.251, -104.292)
  line L6038 (108.554, -105.762) -> (108.535, -105.858)
  line L6039 (106.627, -106.951) -> (103.463, -106.951)
  line L6040 (101.073, -106.852) -> (101.073, -106.902)
  line L6041 (106.862, -106.893) -> (106.814, -106.91)
  line L6042 (103.406, -106.944) -> (103.356, -106.94)
  line L6043 (103.356, -106.94) -> (103.337, -106.933)
  line L6044 (103.369, -105.852) -> (103.42, -105.859)
  line L6045 (103.658, -105.951) -> (106.42, -105.951)
  line L6046 (105.273, -104.012) -> (105.342, -103.889)
  line L6047 (103.463, -106.951) -> (103.457, -106.951)
  line L6048 (103.337, -106.933) -> (103.317, -106.93)
  line L6049 (101.073, -105.802) -> (101.073, -105.852)
  line L6050 (103.619, -105.925) -> (103.638, -105.934)
  line L6051 (103.207, -106.878) -> (103.188, -106.869)
  line L6052 (106.768, -106.931) -> (106.748, -106.934)
  line L6053 (106.935, -106.839) -> (106.897, -106.873)
  line L6054 (106.977, -106.809) -> (106.935, -106.839)
  line L6055 (108.4, -105.993) -> (108.304, -106.012)
  line L6056 (103.42, -105.859) -> (103.471, -105.863)
  line L6057 (96.4732, -105.802) -> (101.073, -105.802)
  line L6058 (103.556, -105.895) -> (103.603, -105.913)
  line L6059 (103.471, -105.863) -> (103.489, -105.87)
  line L6060 (103.363, -105.852) -> (103.369, -105.852)
  line L6061 (103.789, -102.968) -> (103.854, -103.011)
  line L6062 (105.251, -104.292) -> (105.242, -104.151)
  line L6063 (103.897, -103.076) -> (103.913, -103.153)
  line L6064 (107.774, -106.012) -> (106.981, -106.805)
  line L6065 (103.913, -103.153) -> (103.913, -103.553)
  line L6066 (101.073, -106.902) -> (96.4732, -106.902)
  line L6067 (108.535, -105.858) -> (108.481, -105.939)
  line L6068 (105.387, -104.544) -> (105.382, -104.54)
  line L6069 (101.073, -105.852) -> (103.363, -105.852)
  line L6070 (106.878, -106.881) -> (106.862, -106.893)
  line L6071 (105.382, -104.54) -> (105.299, -104.426)
  line L6072 (105.568, -103.722) -> (105.706, -103.692)
  line L6073 (102.978, -103.076) -> (103.021, -103.011)
  line L6074 (105.143, -101.543) -> (105.171, -101.561)
  line L6075 (103.313, -103.753) -> (103.163, -103.753)
  line L6076 (105.372, -101.644) -> (105.496, -101.664)
  line L6077 (103.563, -103.753) -> (103.563, -104.401)
  line L6078 (101.073, -105.202) -> (96.4732, -105.202)
  line L6079 (103.111, -105.186) -> (103.047, -105.143)
  line L6080 (103.563, -104.401) -> (103.738, -104.401)
  line L6081 (103.313, -104.401) -> (103.313, -103.753)
  line L6082 (103.815, -104.417) -> (103.879, -104.46)
  line L6083 (103.738, -105.201) -> (103.188, -105.201)
  line L6084 (103.086, -103.737) -> (103.021, -103.694)
  line L6085 (102.988, -104.852) -> (101.073, -104.852)
  line L6086 (103.938, -105.001) -> (103.923, -105.078)
  line L6087 (102.963, -103.553) -> (102.963, -103.153)
  line L6088 (103.879, -104.46) -> (103.923, -104.525)
  line L6089 (103.815, -105.186) -> (103.738, -105.201)
  line L6090 (101.073, -104.852) -> (101.073, -105.202)
  line L6091 (103.789, -103.737) -> (103.713, -103.753)
  line L6092 (96.4732, -104.102) -> (101.073, -104.102)
  line L6093 (103.188, -104.401) -> (103.313, -104.401)
  line L6094 (102.963, -103.153) -> (102.978, -103.076)
  line L6095 (105.117, -101.523) -> (105.143, -101.543)
  line L6096 (103.923, -104.525) -> (103.938, -104.601)
  line L6097 (105.756, -102.146) -> (105.91, -102.3)
  line L6098 (103.938, -104.601) -> (103.938, -105.001)
  line L6099 (101.073, -104.102) -> (101.073, -104.452)
  line L6100 (103.854, -101.361) -> (103.897, -101.426)
  line L6101 (105.91, -102.3) -> (106.754, -102.3)
  line L6102 (105.03, -101.503) -> (105.063, -101.51)
  line L6103 (103.021, -103.694) -> (102.978, -103.629)
  line L6104 (103.047, -105.143) -> (103.003, -105.078)
  line L6105 (106.754, -102.3) -> (106.754, -102.162)
  line L6106 (103.021, -103.011) -> (103.086, -102.968)
  line L6107 (103.879, -105.143) -> (103.815, -105.186)
  line L6108 (103.059, -104.452) -> (103.111, -104.417)
  line L6109 (103.086, -102.968) -> (103.163, -102.953)
  line L6110 (103.789, -101.318) -> (103.854, -101.361)
  line L6111 (103.111, -104.417) -> (103.188, -104.401)
  line L6112 (102.988, -105.001) -> (102.988, -104.852)
  line L6113 (103.188, -105.201) -> (103.111, -105.186)
  line L6114 (105.772, -102.044) -> (105.756, -102.146)
  line L6115 (103.713, -102.953) -> (103.789, -102.968)
  line L6116 (96.4732, -105.202) -> (96.4732, -104.102)
  line L6117 (103.713, -103.753) -> (103.563, -103.753)
  line L6118 (103.738, -104.401) -> (103.815, -104.417)
  line L6119 (103.003, -105.078) -> (102.988, -105.001)
  line L6120 (103.854, -103.694) -> (103.789, -103.737)
  line L6121 (103.163, -103.753) -> (103.086, -103.737)
  line L6122 (103.923, -105.078) -> (103.879, -105.143)
  line L6123 (103.913, -101.503) -> (105.03, -101.503)
  line L6124 (102.978, -103.629) -> (102.963, -103.553)
  line L6125 (101.073, -104.452) -> (103.059, -104.452)
  line L6126 (105.063, -101.51) -> (105.096, -101.514)
  line L6127 (103.086, -101.318) -> (103.163, -101.303)
  line L6128 (105.254, -90.45) -> (105.366, -90.5068)
  line L6129 (105.511, -90.954) -> (105.454, -91.0655)
  line L6130 (103.163, -101.303) -> (103.713, -101.303)
  line L6131 (102.978, -101.979) -> (102.963, -101.903)
  line L6132 (106.754, -102.7) -> (105.827, -102.7)
  line L6133 (105.686, -102.641) -> (105.473, -102.428)
  line L6134 (105.131, -91.2304) -> (105.007, -91.2108)
  line L6135 (108.481, -101.985) -> (108.535, -102.067)
  line L6136 (108.304, -101.912) -> (108.4, -101.931)
  line L6137 (103.163, -102.953) -> (103.713, -102.953)
  line L6138 (105.714, -102.659) -> (105.686, -102.641)
  line L6139 (106.908, -101.931) -> (107.004, -101.912)
  line L6140 (108.535, -102.067) -> (108.554, -102.162)
  line L6141 (105.372, -102.444) -> (105.248, -102.425)
  line L6142 (108.304, -103.062) -> (107.004, -103.062)
  line L6143 (105.048, -102.28) -> (104.991, -102.168)
  line L6144 (105.096, -101.514) -> (105.106, -101.52)
  line L6145 (105.366, -91.154) -> (105.254, -91.2108)
  line L6146 (105.106, -101.52) -> (105.117, -101.523)
  line L6147 (105.454, -90.5953) -> (105.511, -90.7068)
  line L6148 (104.991, -102.168) -> (104.972, -102.044)
  line L6149 (105.454, -91.0655) -> (105.366, -91.154)
  line L6150 (105.607, -101.721) -> (105.696, -101.809)
  line L6151 (105.473, -102.428) -> (105.372, -102.444)
  line L6152 (103.789, -102.087) -> (103.713, -102.103)
  line L6153 (108.481, -102.989) -> (108.4, -103.043)
  line L6154 (105.74, -102.68) -> (105.714, -102.659)
  line L6155 (105.761, -102.688) -> (105.751, -102.682)
  line L6156 (108.4, -101.931) -> (108.481, -101.985)
  line L6157 (105.271, -101.661) -> (105.372, -101.644)
  line L6158 (107.004, -103.062) -> (106.908, -103.043)
  line L6159 (107.004, -101.912) -> (108.304, -101.912)
  line L6160 (103.713, -102.103) -> (103.163, -102.103)
  line L6161 (105.752, -101.921) -> (105.772, -102.044)
  line L6162 (105.496, -101.664) -> (105.607, -101.721)
  line L6163 (106.827, -101.985) -> (106.908, -101.931)
  line L6164 (108.554, -102.812) -> (108.535, -102.908)
  line L6165 (105.007, -91.2108) -> (104.895, -91.154)
  line L6166 (105.171, -101.561) -> (105.271, -101.661)
  line L6167 (103.713, -101.303) -> (103.789, -101.318)
  line L6168 (105.366, -90.5068) -> (105.454, -90.5953)
  line L6169 (105.794, -102.692) -> (105.761, -102.688)
  line L6170 (108.535, -102.908) -> (108.481, -102.989)
  line L6171 (105.248, -102.425) -> (105.137, -102.368)
  line L6172 (108.4, -103.043) -> (108.304, -103.062)
  line L6173 (102.963, -101.503) -> (102.978, -101.426)
  line L6174 (106.754, -102.812) -> (106.754, -102.7)
  line L6175 (105.751, -102.682) -> (105.74, -102.68)
  line L6176 (106.827, -102.989) -> (106.773, -102.908)
  line L6177 (106.908, -103.043) -> (106.827, -102.989)
  line L6178 (108.554, -102.162) -> (108.554, -102.812)
  line L6179 (103.897, -101.426) -> (103.913, -101.503)
  line L6180 (106.773, -102.067) -> (106.827, -101.985)
  line L6181 (105.137, -102.368) -> (105.048, -102.28)
  line L6182 (106.773, -102.908) -> (106.754, -102.812)
  line L6183 (104.947, -101.903) -> (103.913, -101.903)
  line L6184 (105.696, -101.809) -> (105.752, -101.921)
  line L6185 (106.754, -102.162) -> (106.773, -102.067)
  line L6186 (105.531, -90.8304) -> (105.511, -90.954)
  line L6187 (105.827, -102.7) -> (105.794, -102.692)
  line L6188 (104.988, -101.943) -> (104.947, -101.903)
  line L6189 (103.913, -101.903) -> (103.897, -101.979)
  line L6190 (102.978, -101.426) -> (103.021, -101.361)
  line L6191 (103.492, -90.6633) -> (103.522, -90.6546)
  line L6192 (104.75, -90.954) -> (104.742, -90.9046)
  line L6193 (102.202, -94.7712) -> (102.201, -94.7737)
  line L6194 (103.163, -102.103) -> (103.086, -102.087)
  line L6195 (102.202, -94.7666) -> (102.202, -94.7712)
  line L6196 (102.201, -94.7737) -> (102.2, -94.7801)
  line L6197 (92.0395, -99.5863) -> (92.0136, -99.5696)
  line L6198 (97.4466, -99.5548) -> (97.4288, -99.5681)
  line L6199 (97.3877, -99.5827) -> (97.3582, -99.5914)
  line L6200 (101.96, -92.1858) -> (101.977, -92.16)
  line L6201 (102.205, -94.7446) -> (102.202, -94.7666)
  line L6202 (104.807, -90.5953) -> (104.895, -90.5068)
  line L6203 (91.4719, -94.7608) -> (91.3604, -94.8176)
  line L6204 (103.433, -90.6912) -> (103.451, -90.6779)
  line L6205 (101.958, -92.1993) -> (101.958, -92.1947)
  line L6206 (97.3582, -99.5914) -> (92.075, -99.5914)
  line L6207 (102.963, -101.903) -> (102.963, -101.503)
  line L6208 (103.454, -90.6744) -> (103.457, -90.6736)
  line L6209 (103.021, -101.361) -> (103.086, -101.318)
  line L6210 (102.2, -94.7801) -> (102.183, -94.806)
  line L6211 (104.807, -91.0655) -> (104.75, -90.954)
  line L6212 (101.958, -92.1947) -> (101.959, -92.1922)
  line L6213 (103.451, -90.6779) -> (103.454, -90.6744)
  line L6214 (92.075, -99.5914) -> (92.053, -99.5882)
  line L6215 (91.3604, -94.8176) -> (91.2368, -94.8372)
  line L6216 (97.3064, -99.3414) -> (101.955, -94.6928)
  line L6217 (97.4288, -99.5681) -> (97.4257, -99.5716)
  line L6218 (103.854, -102.044) -> (103.789, -102.087)
  line L6219 (105.511, -90.7068) -> (105.531, -90.8304)
  line L6220 (97.423, -99.5724) -> (97.4178, -99.5763)
  line L6221 (92.0484, -99.5885) -> (92.0459, -99.5872)
  line L6222 (90.9132, -94.6723) -> (90.8999, -94.6461)
  line L6223 (104.895, -90.5068) -> (105.007, -90.45)
  line L6224 (103.021, -102.044) -> (102.978, -101.979)
  line L6225 (103.522, -90.6546) -> (104.777, -90.6546)
  line L6226 (92.0136, -99.5696) -> (91.9866, -99.5548)
  line L6227 (92.053, -99.5882) -> (92.0484, -99.5885)
  line L6228 (90.8999, -94.6461) -> (90.1172, -95.4288)
  line L6229 (102.205, -92.2731) -> (102.205, -94.7446)
  line L6230 (103.574, -90.9046) -> (102.205, -92.2731)
  line L6231 (104.972, -102.044) -> (104.988, -101.943)
  line L6232 (104.895, -91.154) -> (104.807, -91.0655)
  line L6233 (90.1172, -95.4288) -> (90.1172, -97.3318)
  line L6234 (102.183, -94.806) -> (102.168, -94.833)
  line L6235 (101.959, -92.1922) -> (101.96, -92.1858)
  line L6236 (101.977, -92.16) -> (101.992, -92.133)
  line L6237 (104.777, -90.6546) -> (104.807, -90.5953)
  line L6238 (103.897, -101.979) -> (103.854, -102.044)
  line L6239 (102.168, -94.833) -> (97.4466, -99.5548)
  line L6240 (90.1172, -97.3318) -> (92.1268, -99.3414)
  line L6241 (97.4178, -99.5763) -> (97.3877, -99.5827)
  line L6242 (92.0459, -99.5872) -> (92.0395, -99.5863)
  line L6243 (101.955, -94.6928) -> (101.955, -92.2213)